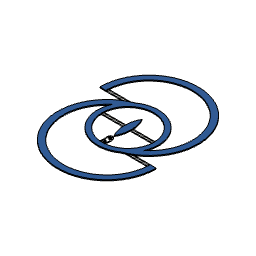
キキョウ_ヘイロー_mk1 v1 (Autodesk Fusion 360 design; units mm, degrees)
Autodesk Fusion 360 part; units mm, degrees
sketch "スケッチ1" plane through (0, 0, 0) normal (0, 0, 1) x (1, 0, 0)
  line L0 (0, 0) -> (0, -100) construction
  circle A0 centre (0, -45) radius 55
  arc A1 (-59.7357, -19.375) -> (92.5, -90) centre (0, -90) ccw
  arc A2 (-37.5514, 8.0556) -> (105, -90) centre (0, -90) ccw
  arc A3 (59.7357, -70.625) -> (-92.5, 0) centre (0, 0) ccw
  arc A4 (37.5514, -98.0556) -> (-105, 0) centre (0, 0) ccw
  line L1 (0, 0) -> (-92.5, 0) construction
  line L2 (-92.5, 0) -> (-105, 0)
  line L3 (0, -90) -> (92.5, -90) construction
  line L4 (92.5, -90) -> (105, -90)
  arc A5 (59.7357, -70.625) -> (-37.5514, 8.0556) centre (0, -45) ccw
  arc A6 (-59.7357, -19.375) -> (37.5514, -98.0556) centre (0, -45) ccw
  line L5 (-7.5, -45) -> (7.5, -45) construction
  arc A7 (0, -15) -> (0, -75) centre (56.25, -45) ccw
  arc A8 (0, -75) -> (0, -15) centre (-56.25, -45) ccw
  line L6 (-54.9432, -42.5) -> (-7.451, -42.5)
  line L7 (-54.9432, -47.5) -> (-7.451, -47.5)
  line L8 (54.9432, -42.5) -> (7.451, -42.5)
  line L9 (54.9432, -47.5) -> (7.451, -47.5)
  line L10 (-92.5, 0) -> (-54.0833, 0)
  line L11 (-92.3648, 5) -> (-44.7214, 5)
  line L12 (92.5, -90) -> (54.0833, -90)
  line L13 (92.3648, -95) -> (44.7214, -95)
  circle A9 centre (0, -83) radius 2.6
  circle A10 centre (0, -95) radius 2.6
  line L14 (-5, -83) -> (-5, -99.7723)
  line L15 (5, -83) -> (5, -99.7723)
  arc A11 (0, -78) -> (-5, -83) centre (0, -83) ccw
  arc A12 (5, -83) -> (0, -78) centre (0, -83) ccw
  point P0 (0, -15)
  point P1 (0, -75)
  point P2 (-5, -78)
  point P3 (5, -78)
  dimension "d1" = 210
  dimension "d2" = 185
  dimension "d3" = 90
  dimension "d4" = 210
  dimension "d5" = 185
  dimension "d6" = 130
  dimension "d7" = 110
  dimension "d8" = 15
  dimension "d9" = 30
  dimension "d10" = 30
  dimension "d11" = 5
  dimension "d12" = 5
  dimension "d13" = 5
  dimension "d14" = 5.2
  dimension "d15" = 5.2
  dimension "d16" = 12
  dimension "d17" = 5
  dimension "d18" = 10
  dimension "d24" = 5
  constraint coincident L0.start A3.centre
  constraint concentric A3 A4
  constraint vertical L0
  constraint concentric A1 A2
  constraint concentric A0 A5
  constraint coincident A1.start A5
  constraint horizontal L1
  constraint parallel L1 L2
  constraint coincident A1.centre A2.centre
  constraint perpendicular L0 L3
  constraint parallel L3 L4
  constraint concentric A5 A6
  constraint perpendicular L0 L5
  constraint midpoint A0.centre L5
  constraint coincident L0 P0
  constraint coincident L0 P1
  constraint coincident L5.start A7
  constraint coincident P1 A7.end
  constraint coincident P0 A7.start
  constraint coincident L5.end A8
  constraint coincident A0 L6.start
  constraint coincident A7 L6.end
  constraint coincident A7 L7.end
  constraint parallel L6 L7
  constraint coincident A0 L7.start
  constraint symmetric L5 L6 L7
  constraint symmetric L0 L6.start L8.start
  constraint symmetric L0 L6.end L8.end
  constraint symmetric L0 L7.start L9.start
  constraint symmetric L0 L7.end L9.end
  constraint coincident A2 L10.end
  constraint coincident L1 L10.end
  constraint coincident A3 L11.start
  constraint coincident A2 L11.end
  constraint parallel L10 L11
  constraint coincident A4 L12.end
  constraint coincident L3 L12.end
  constraint coincident A1 L13.start
  constraint coincident A4 L13.end
  constraint parallel L12 L13
  constraint coincident L0 A9.centre
  constraint coincident L0 A0.centre
  constraint coincident A0 L0.end
  constraint coincident A0 L14.end
  constraint coincident A0 L15.end
  constraint coincident P2 L14
  constraint tangent L14 A11
  constraint coincident P3 L15
  constraint tangent L15 A12
  constraint equal A11 A12
  constraint coincident A11.start A12.end
  measures "d1" diameter of A4
  measures "d2" diameter of A3
  measures "d3" distance of L0.start A1.centre
  measures "d4" diameter of A2
  measures "d5" diameter of A1
  measures "d6" diameter of A5
  measures "d7" diameter of A0
  measures "d8" distance of L5.start L5.end
  measures "d9" distance of A0.centre P0
  measures "d10" distance of A0.centre P1
  measures "d11" distance of L6 L7
  measures "d12" distance of L10 L11
  measures "d13" distance of L12 L13
  measures "d14" diameter of A9
  measures "d15" diameter of A10
  measures "d16" distance of A9.centre A10.centre
  measures "d17" distance of A10.centre L0.end
  measures "d18" distance of P2 P3
  measures "d24" radius of A11
extrude "押し出し1" add sketch "スケッチ1" along normal blind 2 contours A7 A8 | A1 A2 A3 A4 L2 L4 A5 A6 makes body 1 at (54.0161, -83.3084, 2) makes body 2 at (2.0332, -37.5983, 0)
extrude "押し出し2" add sketch "スケッチ1" along normal blind 2 separate body contours A0 A8 L8 L9 | A0 A7 L6 L7 | A0 L14 L15 A11 A12 | A1 A4 L12 L13 | A2 A3 L10 L11 makes body 3 at (-4.1903, -92.4616, 2) makes body 4 at (-65.8225, 2.2572, 0) makes body 5 at (65.8225, -92.2572, 0) makes body 6 at (39.1438, -46.389, 2) makes body 7 at (-39.1438, -46.389, 0)
equation "d4 = d1"
equation "d5 = d2"
equation "d10 = d9"
